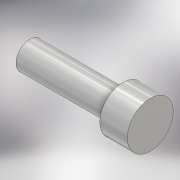
# Autodesk Inventor part: thin nuts
Saved by Autodesk Inventor 2020 (Build 240168000, 168)
## iProperties
Created: 2018-05-08
Part Number: thin nuts
Material: Generic
Document SubType Name: Modeling
Designer: PC  USER
Density: 1 g/cm^3
Appearance: Default
Author: PC  USER
Autodesk Inventor part; units mm, degrees
ref_plane "YZ Plane" through (0, 0, 0) normal (1, 0, 0) x (0, 1, 0)
ref_plane "XZ Plane" through (0, 0, 0) normal (0, 1, 0) x (-1, 0, 0)
ref_plane "XY Plane" through (0, 0, 0) normal (0, 0, 1) x (1, 0, 0)
sketch "Sketch1" plane through (0, 0, 0) normal (0, 1, 0) x (-1, 0, 0)
  line L0 (0, 0) -> (5.9, 0)
  line L1 (5.9, 0) -> (5.9, -4.93)
  line L2 (5.9, -4.93) -> (0, -4.93)
  line L3 (0, -4.93) -> (0, 0)
  line L4 (5.9, 0) -> (25.9, 0)
  line L5 (25.9, 0) -> (25.9, -2.96)
  line L6 (25.9, -2.96) -> (5.9, -2.96)
  line L7 (5.9, -2.96) -> (5.9, 0)
  dimension "d0" = 4.93
  dimension "d1" = 2.96
  dimension "d2" = 5.9
  dimension "d3" = 20
  constraints: 16 end point, 4 parallel, 2 horizontal, 2 perpendicular
  measures "d0" distance of L2.end L0.start
  measures "d1" distance of L4.end L5.end
  measures "d2" distance of L1.end L2.end
  measures "d3" distance of L5.end L6.end
revolve "Revolution1" add sketch "Sketch1" angle 360 about axis through (-5.9, 0, 0) along (-1, 0, 0)
body "Solid1"
